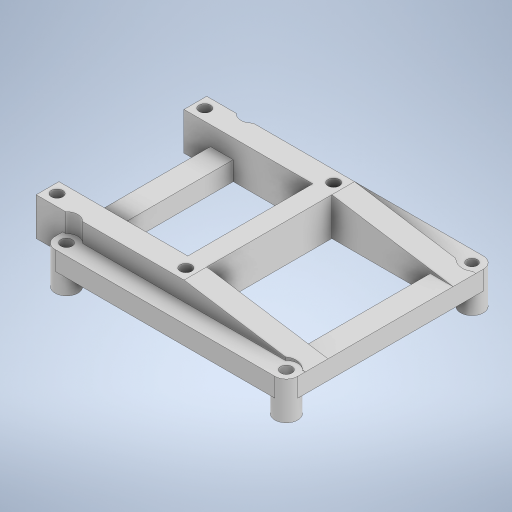
# Autodesk Inventor part: Houder_RPI_v2
Saved by Autodesk Inventor 2023 (Build 270158000, 158)
## iProperties
Created: 2022-12-06
Part Number: Houder_RPI_v2
Material: Generic
Document SubType Name: Modeling
Designer: semih
Density: 1 g/cm^3
Appearance: Default
Author: semih
Autodesk Inventor part; units mm, degrees
ref_plane "YZ Plane" through (0, 0, 0) normal (1, 0, 0) x (0, 1, 0)
ref_plane "XY Plane" through (0, 0, 0) normal (0, 0, 1) x (1, 0, 0)
sketch "Sketch1" plane through (0, 0, 0) normal (0, 1, 0) x (-1, 0, 0)
  circle A0 centre (0, 0) radius 1.5
  circle A1 centre (0, 0) radius 3
  circle A2 centre (-58, 0) radius 1.5
  circle A3 centre (-58, 0) radius 3
  circle A4 centre (0, -49) radius 1.375
  circle A5 centre (0, -49) radius 3
  circle A6 centre (-58, -49) radius 1.375
  circle A7 centre (-58, -49) radius 3
  dimension "d0" = 3
  dimension "d1" = 6
  dimension "d2" = 3
  dimension "d3" = 6
  dimension "d4" = 58
  dimension "d5" = 2.75
  dimension "d6" = 6
  dimension "d9" = 49
  dimension "d10" = 2.75
  dimension "d11" = 6
  constraints: 8 centre point, 5 coincident, 2 horizontal alignment, 2 vertical alignment
  measures "d0" diameter of A0
  measures "d1" diameter of A1
  measures "d2" diameter of A2
  measures "d3" diameter of A3
  measures "d4" distance of A2.centre point (0, 0)
  measures "d5" diameter of A4
  measures "d6" diameter of A5
  measures "d9" distance of A4.centre point (0, 0)
  measures "d10" diameter of A6
  measures "d11" diameter of A7
extrude "Extrusion1" add sketch "Sketch1" along normal blind 10
ref_plane "Work Plane1" through (0, 5, 0) normal (0, 1, 0) x (-1, 0, 0)
sketch "Sketch2" plane through (0, 5, 0) normal (0, 1, 0) x (-1, 0, 0)
  circle A0 centre (0, -49) radius 3 projected
  circle A1 centre (0, 0) radius 3 projected
  circle A2 centre (-58, 0) radius 3 projected
  circle A3 centre (-58, -49) radius 3 projected
  circle A4 centre (0, -49) radius 3 projected
  circle A5 centre (0, 0) radius 3 projected
  circle A6 centre (-58, -49) radius 3 projected
  circle A7 centre (0, -49) radius 1.375 projected
  circle A8 centre (-58, 0) radius 1.5 projected
  line L0 (3, -49) -> (3, 0)
  line L1 (0, -52) -> (-58, -52)
  line L2 (-61, -49) -> (-61, 0)
  circle A9 centre (-58, 0) radius 3 projected
  line L3 (-58, 3) -> (0, 3)
  line L4 (-3, -49) -> (-3, 0)
  line L5 (0, -46) -> (-58, -46)
  line L6 (-55, -49) -> (-55, 0)
  line L7 (-58, -3) -> (0, -3)
  line L8 (-55, -47) -> (-3, -47)
  line L9 (-55, -41) -> (-3, -41)
  line L10 (-55, -8) -> (-3, -8)
  line L11 (-55, -2) -> (-3, -2)
  line L12 (0, -46) -> (10, -46)
  line L13 (10, -46) -> (10, -41)
  line L14 (10, -41) -> (-3, -41)
  line L15 (-3, -8) -> (10, -8)
  line L16 (10, -8) -> (10, -3)
  line L17 (0, -3) -> (10, -3)
  line L18 (10, -41) -> (10, -8)
  line L19 (5, -41) -> (5, -8)
  line L20 (-24, -46) -> (-24, -8)
  line L21 (-29, -46) -> (-29, -8)
  point P0 (-3, -46)
  point P1 (-55, -46)
  point P2 (-55, -3)
  point P3 (-3, -3)
  point P4 (3, 0)
  point P5 (0, 3)
  point P6 (-61, 0)
  point P7 (-44, -3)
  point P8 (-39, -3)
  point P9 (3, -3)
  point P10 (3, -8)
  point P11 (-24, -41)
  point P12 (-29, -41)
  dimension "d23" = -1
  dimension "d25" = -1
  dimension "d45" = 39
  dimension "d46" = 10
  dimension "d47" = 5
  dimension "d48" = 34
  dimension "d49" = 5
  dimension "d77" = 5
  dimension "d78" = 5
  constraints: 44 end point, 18 point on line, 18 tangent, 15 point on circle, 10 perpendicular, 2 midpoint, 2 parallel, 1 horizontal, 1 vertical, 2 other
  measures "d23" distance between parallel lines of L5 L8
  measures "d25" distance between parallel lines of L7 L11
  measures "d45" distance between parallel lines of L11 L9
  measures "d46" distance of L5.start L12.end
  measures "d47" distance between parallel lines of L19 L18
  measures "d48" distance between parallel lines of L18 L20
  measures "d49" distance between parallel lines of L20 L21
  measures "d77" distance between parallel lines of L7 L10
  measures "d78" distance between parallel lines of L9 L5
extrude "Extrusion2" add sketch "Sketch2" along normal up to surface (5 mm away) contours A0 L12 L0 | A0 L4 L5 | L5 L4 L14 L0 L12 | L1 A3 L6 L8 L4 A0 | L0 L14 L13 L12 | L5 L20 L9 L4 | L14 L4 L15 L0 | L5 L21 L9 L20 | L2 A2 L7 L6 L5 A3 | A3 L5 L6 | L15 L4 L7 L17 L0 | L0 L17 L16 L15 | L19 L15 L18 L14 | L10 L6 L7 L4 | L9 L21 L10 L20 | L5 L6 L9 L21 | L17 A1 L0 | L4 A1 L7 | L3 A1 L4 L11 L6 A2 | A2 L6 L7
sketch "Sketch8" plane through (-10, 5, -3) normal (0, 0, 1) x (1, 0, 0)
  line L0 (7, 5) -> (0, 5) projected
  line L1 (10, 5) -> (7, 5) projected
  line L2 (68, 5) -> (10, 5) projected
  line L3 (71, 5) -> (68, 5) projected
  line L4 (39, 0) -> (39, 5) projected
  line L5 (39, 5) -> (39, 10)
  line L6 (39, 10) -> (71, 5)
  line L7 (0, 5) -> (7, 5) projected
  line L8 (0, 5) -> (0, 10)
  line L9 (0, 10) -> (39, 10)
  point P0 (10, -5)
  dimension "d50" = 5
  dimension "d51" = 5
  constraints: 8 end point, 2 vertical
  measures "d50" distance of L4.end L5.end
  measures "d51" distance of L0.end L8.end
extrude "Extrusion8" add sketch "Sketch8" against normal up to surface (5 mm away)
sketch "Sketch9" plane through (-3, 5, -46) normal (0, 0, -1) x (-1, 0, 0)
  line L0 (-32, 10) -> (7, 10) projected
  line L1 (-64, 5) -> (-32, 10) projected
  line L2 (-58, 5) -> (-64, 5) projected
  line L3 (-3, 5) -> (-61, 5) projected
  line L4 (0, 5) -> (-3, 5) projected
  line L5 (7, 5) -> (0, 5) projected
  line L6 (7, 10) -> (7, 5) projected
  point P0 (-3, -5)
extrude "Extrusion9" add sketch "Sketch9" against normal up to surface (5 mm away)
sketch "Sketch10" plane through (-10, 5, -46) normal (-1, 0, 0) x (0, 0, 1)
  line L0 (38, 5) -> (5, 5) projected
  line L1 (5, 5) -> (5, 10) projected
  line L2 (0, 10) -> (5, 10) projected
  line L3 (0, 0) -> (0, 10) projected
  line L4 (0, 0) -> (43, 0) projected
  line L5 (43, 0) -> (43, 10) projected
  line L6 (43, 10) -> (38, 10) projected
  line L7 (38, 10) -> (38, 5) projected
  line L8 (0, 10) -> (5, 10) projected
  line L9 (5, 10) -> (38, 10)
  point P0 (46, -5)
  constraints: 2 end point, 1 horizontal
extrude "Extrusion10" add sketch "Sketch10" against normal up to surface (5 mm away) contours L0 L1 L9 L7
sketch "Sketch11" plane through (29, 5, -8) normal (1, 0, 0) x (0, 0, -1)
  line L0 (0, 10) -> (33, 10) projected
  line L1 (33, 5) -> (0, 5) projected
  line L2 (0, 0) -> (0, 10) projected
  line L3 (33, 0) -> (33, 10) projected
  point P0 (-8, -5)
extrude "Extrusion11" add sketch "Sketch11" against normal up to surface (5 mm away)
sketch "Sketch12" plane through (-10, 15, -3) normal (0, 1, 0) x (1, 0, 0)
  circle A0 centre (2.5, 2) radius 1.5
  circle A1 centre (2.5, 41) radius 1.5
  line L0 (0, 43) -> (0, 0) projected
  line L1 (39, 0) -> (0, 0) projected
  line L2 (0, 43) -> (39, 43) projected
  circle A2 centre (36.5, 2) radius 1.5
  circle A3 centre (36.5, 41) radius 1.5
  line L3 (39, 38) -> (39, 5) projected
  line L4 (5, 38) -> (34, 38) projected
  line L5 (34, 5) -> (5, 5) projected
  point P0 (10, -3)
  dimension "d60" = 3
  dimension "d61" = 3
  dimension "d62" = 2.5
  dimension "d64" = 2.5
  dimension "d66" = 3
  dimension "d67" = 3
  dimension "d69" = 2.5
  dimension "d70" = 2.5
  dimension "d79" = 39
  dimension "d80" = 39
  dimension "d81" = 3
  dimension "d82" = 3
  dimension "d83" = 3
  dimension "d84" = 3
  constraints: 4 centre point
  measures "d60" diameter of A0
  measures "d61" diameter of A1
  measures "d62" distance from line of L0 A0.centre
  measures "d64" distance from line of L0 A1.centre
  measures "d66" diameter of A2
  measures "d67" diameter of A3
  measures "d69" distance from line of L3 A2.centre
  measures "d70" distance from line of L3 A3.centre
  measures "d79" distance of A2.centre A3.centre
  measures "d80" distance of A0.centre A1.centre
  measures "d81" distance from line of L4 A3.centre
  measures "d82" distance from line of L5 A2.centre
  measures "d83" distance from line of L4 A1.centre
  measures "d84" distance from line of L5 A0.centre
extrude "Extrusion12" cut sketch "Sketch12" against normal up to surface (10 mm away)
sketch "Sketch13" plane through (-10, 5, -46) normal (-1, 0, 0) x (0, 0, 1)
  line L0 (5, 0) -> (5, 10) projected
  line L1 (38, 0) -> (38, 10) projected
  line L2 (0, 10) -> (43, 10) projected
  line L3 (0, 0) -> (43, 0) projected
  point P0 (46, -5)
extrude "Extrusion13" cut sketch "Sketch13" against normal blind 5
sketch "Sketch14" plane through (55, 5, -46) normal (0, 0, -1) x (-1, 0, 0)
  line L0 (0, 0) -> (0, 5) projected
  line L1 (0, 0) -> (52, 0) projected
  line L2 (52, 0) -> (52, 5) projected
  line L3 (58, 5) -> (52, 5) projected
  line L4 (58, 0) -> (58, 5) projected
  line L5 (58, 0) -> (65, 0) projected
  line L6 (65, 0) -> (65, 10) projected
  line L7 (65, 10) -> (26, 10) projected
  line L8 (26, 10) -> (-6, 5) projected
  line L9 (0, 5) -> (-6, 5) projected
  point P0 (55, -5)
extrude "Extrusion14" add sketch "Sketch14" along normal up to surface (1 mm away)
sketch "Sketch15" plane through (3, 5, -3) normal (0, 0, 1) x (1, 0, 0)
  line L0 (0, 0) -> (0, 5) projected
  line L1 (0, 0) -> (52, 0) projected
  line L2 (52, 0) -> (52, 5) projected
  line L3 (58, 5) -> (52, 5) projected
  line L4 (58, 5) -> (26, 10) projected
  line L5 (26, 10) -> (-13, 10) projected
  line L6 (-13, 0) -> (-13, 10) projected
  line L7 (-13, 0) -> (-6, 0) projected
  line L8 (-6, 0) -> (-6, 5) projected
  line L9 (0, 5) -> (-6, 5) projected
  point P0 (-3, -5)
extrude "Extrusion15" add sketch "Sketch15" along normal up to surface (1 mm away)
sketch "Sketch16" plane through (0, 10, 0) normal (0, 1, 0) x (1, 0, 0)
  circle A0 centre (0, 0) radius 1.5 projected
  circle A1 centre (0, 0) radius 3
  circle A2 centre (0, 49) radius 1.375 projected
  circle A3 centre (0, 49) radius 3
  circle A4 centre (58, 49) radius 1.375 projected
  circle A5 centre (58, 49) radius 3
  circle A6 centre (58, 0) radius 1.5 projected
  circle A7 centre (58, 0) radius 3
  constraints: 4 centre point, 4 coincident
extrude "Extrusion16" cut sketch "Sketch16" along normal up to surface (5 mm away)
equation "\"d2\" = d0"
equation "\"d3\" = d1"
equation "\"d5\" = d7"
equation "\"d6\" = d8"
equation "\"d10\" = d12"
equation "\"d11\" = d13"
equation "\"d23\" = d25"
equation "\"d47\" = d21"
equation "\"d49\" = d21"
equation "\"d51\" = d50"
equation "\"d61\" = d60"
equation "\"d66\" = d60"
equation "\"d67\" = d60"
equation "\"d80\" = d79"
equation "\"d81\" = d82"
equation "\"d83\" = d82"
equation "\"d7\" = 2.75"
equation "\"d8\" = 6"
equation "\"d12\" = 2.75"
equation "\"d13\" = 6"
equation "\"d21\" = 5"
body "Solid1"
